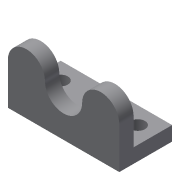
# Autodesk Inventor part: Guide Bracket
Saved by Autodesk Inventor 2022 (Build 260148000, 148)
## iProperties
Created: 2009-04-22
Part Number: Guide Bracket
Document SubType Name: Modeling
Designer: esverko
Density: 1 g/cm^3
Material: Generic
Mass: 44.7642 g
Surface Area: 142.663 cm^2
Volume: 44.7642 cm^3
Appearance: Default
d19: 0.00 deg
d5: 12.000 mm
d6: 12.000 mm
d7: 10.000 mm
d8: 0.00 deg
d9: 10.000 mm
d10: 60.000 mm
d11: 0.00 deg
d0: 78.000 mm
d1: 37.000 mm
d2: 10.000 mm
d3: 12.000 mm
d4: 12.000 mm
d12: 6.000 mm
d13: 26.000 mm
Author: esverko
Autodesk Inventor part; units mm, degrees
ref_plane "YZ Plane" through (0, 0, 0) normal (1, 0, 0) x (0, 1, 0)
ref_plane "XZ Plane" through (0, 0, 0) normal (0, 1, 0) x (-1, 0, 0)
ref_plane "XY Plane" through (0, 0, 0) normal (0, 0, 1) x (1, 0, 0)
sketch "Sketch1" plane through (0, 0, 0) normal (0, 0, 1) x (1, 0, 0)
  line L0 (0, 37) -> (-78, 37)
  line L1 (-78, 37) -> (-78, 0)
  line L2 (-78, 0) -> (0, 0)
  line L3 (0, 0) -> (0, 37)
  circle A0 centre (-12, 25) radius 5
  circle A1 centre (-66, 25) radius 5
  point P0 (-39, 0)
  dimension "d0" = 78
  dimension "d1" = 37
  dimension "d2" = 10
  dimension "d3" = 12
  dimension "d4" = 12
  dimension "d5" = 12
  dimension "d6" = 12
  constraints: 8 end point, 2 centre point, 2 parallel, 1 coincident, 1 equal radius, 1 horizontal, 1 midpoint, 1 perpendicular
  measures "d0" distance of L0.start L0.end
  measures "d1" distance of L2.end L0.start
  measures "d2" diameter of A0
  measures "d3" horizontal distance of L0.start A0.centre
  measures "d4" horizontal distance of L0.start A0.centre
  measures "d5" horizontal distance of L0.end A1.centre
  measures "d6" horizontal distance of L0.end A1.centre
extrude "Extrusion1" add sketch "Sketch1" along normal blind 10
sketch "Sketch2" plane through (0, 0, 10) normal (0, 0, 1) x (1, 0, 0)
  line L0 (0, 37) -> (0, 0) projected
  line L1 (-78, 0) -> (-78, 37) projected
  line L2 (0, 0) -> (-78, 0) projected
  line L3 (0, 10) -> (-78, 10)
  dimension "d9" = 10
  constraints: 2 end point, 2 point on line, 1 parallel
  measures "d9" distance of L0.end L3.start
extrude "Extrusion2" add sketch "Sketch2" along normal blind 60 separate body
sketch "Sketch4" plane through (-78, 10, 10) normal (0, 1, 0) x (1, 0, 0)
  line L0 (0, -60) -> (78, -60) projected
  line L1 (78, 0) -> (78, -60) projected
  line L2 (0, 0) -> (0, -60) projected
  line L3 (78, -32) -> (52, -32)
  line L4 (52, -32) -> (52, -6)
  line L5 (52, -6) -> (26, -6)
  line L6 (26, -6) -> (26, -32)
  line L7 (26, -32) -> (0, -32)
  point P0 (78, 10)
  dimension "d12" = 6
  dimension "d13" = 26
  constraints: 10 end point, 4 parallel, 3 perpendicular, 2 point on line, 1 collinear
  measures "d12" vertical distance of L1.start L4.end
  measures "d13" distance of L4.end L3.end
extrude "Extrusion4" cut sketch "Sketch4" against normal through all bodies 2
full round fillet "Fillet4" bodies 2 first side at (0, 6.6667, 31.3333) centre faces at (-8.6667, 6.6667, 42) second side at (-26, 6.6667, 33.3333)
full round fillet "Fillet5" bodies 2 first side at (-52, 6.6667, 24.6667) centre faces at (-60.6667, 3.3333, 42) second side at (-78, 3.3333, 31.3333)
full round fillet "Fillet6" bodies 2 first side at (-52, 6.6667, 20.3334) centre faces at (-34.6667, 3.3333, 16) second side at (-26, 3.3333, 24.6667)
body "Solid1"
body "Solid2"
